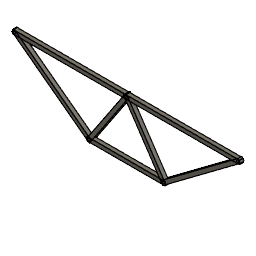
Truss_Assembly (Autodesk Fusion 360 design; units mm, degrees)
part number: 2026-09-01-19-27-21-433
Autodesk Fusion 360 part; units mm, degrees
sketch "Sketch1" plane through (0, 0, 0) normal (0, 0, 1) x (1, 0, 0)
  line L0 (-10.5, -10.5) -> (10.5, -10.5)
  line L1 (10.5, -10.5) -> (10.5, 10.5)
  line L2 (10.5, 10.5) -> (-10.5, 10.5)
  line L3 (-10.5, 10.5) -> (-10.5, -10.5)
sketch "Sketch2" plane through (0, 0, 0) normal (0, 0, 1) x (1, 0, 0)
  line L0 (-10.5, -10.5) -> (10.5, -10.5)
  line L1 (10.5, -10.5) -> (10.5, 10.5)
  line L2 (10.5, 10.5) -> (-10.5, 10.5)
  line L3 (-10.5, 10.5) -> (-10.5, -10.5)
sketch "Sketch3" plane through (0, 0, 0) normal (0, 0, 1) x (1, 0, 0)
  line L0 (-10.5, -10.5) -> (10.5, -10.5)
  line L1 (10.5, -10.5) -> (10.5, 10.5)
  line L2 (10.5, 10.5) -> (-10.5, 10.5)
  line L3 (-10.5, 10.5) -> (-10.5, -10.5)
sketch "Sketch4" plane through (0, 0, 0) normal (0, 0, 1) x (1, 0, 0)
  line L0 (-10.5, -10.5) -> (10.5, -10.5)
  line L1 (10.5, -10.5) -> (10.5, 10.5)
  line L2 (10.5, 10.5) -> (-10.5, 10.5)
  line L3 (-10.5, 10.5) -> (-10.5, -10.5)
sketch "Sketch5" plane through (0, 0, 0) normal (0, 0, 1) x (1, 0, 0)
  line L0 (-10.5, -10.5) -> (10.5, -10.5)
  line L1 (10.5, -10.5) -> (10.5, 10.5)
  line L2 (10.5, 10.5) -> (-10.5, 10.5)
  line L3 (-10.5, 10.5) -> (-10.5, -10.5)
sketch "Sketch6" plane through (0, 0, 0) normal (0, 0, 1) x (1, 0, 0)
  line L0 (-10.5, -10.5) -> (10.5, -10.5)
  line L1 (10.5, -10.5) -> (10.5, 10.5)
  line L2 (10.5, 10.5) -> (-10.5, 10.5)
  line L3 (-10.5, 10.5) -> (-10.5, -10.5)
sketch "Sketch7" plane through (0, 0, 0) normal (0, 0, 1) x (1, 0, 0)
  line L0 (-10.5, -10.5) -> (10.5, -10.5)
  line L1 (10.5, -10.5) -> (10.5, 10.5)
  line L2 (10.5, 10.5) -> (-10.5, 10.5)
  line L3 (-10.5, 10.5) -> (-10.5, -10.5)
sketch "Sketch8" plane through (0, 0, 0) normal (0, 0, 1) x (1, 0, 0)
  circle A0 centre (0, 0) radius 6.25
sketch "Sketch9" plane through (0, 0, 0) normal (0, 0, 1) x (1, 0, 0)
  circle A0 centre (600, 0) radius 6.25
sketch "Sketch10" plane through (0, 0, 0) normal (0, 0, 1) x (1, 0, 0)
  circle A0 centre (1200, 0) radius 6.25
sketch "Sketch11" plane through (0, 0, 0) normal (0, 0, 1) x (1, 0, 0)
  circle A0 centre (400, -299.3326) radius 6.25
sketch "Sketch12" plane through (0, 0, 0) normal (0, 0, 1) x (1, 0, 0)
  circle A0 centre (800, -299.3326) radius 6.25
sketch "Sketch13" plane through (0, 0, 0) normal (0, 0, 1) x (1, 0, 0)
  circle A0 centre (0, 0) radius 6.25
sketch "Sketch14" plane through (0, 0, 0) normal (0, 0, 1) x (1, 0, 0)
  circle A0 centre (0, 0) radius 6.25
sketch "Sketch15" plane through (0, 0, 0) normal (0, 0, 1) x (1, 0, 0)
  circle A0 centre (600, 0) radius 6.25
sketch "Sketch16" plane through (0, 0, 0) normal (0, 0, 1) x (1, 0, 0)
  circle A0 centre (600, 0) radius 6.25
sketch "Sketch17" plane through (0, 0, 0) normal (0, 0, 1) x (1, 0, 0)
  circle A0 centre (1200, 0) radius 6.25
sketch "Sketch18" plane through (0, 0, 0) normal (0, 0, 1) x (1, 0, 0)
  circle A0 centre (1200, 0) radius 6.25
sketch "Sketch19" plane through (0, 0, 0) normal (0, 0, 1) x (1, 0, 0)
  circle A0 centre (400, -299.3326) radius 6.25
sketch "Sketch20" plane through (0, 0, 0) normal (0, 0, 1) x (1, 0, 0)
  circle A0 centre (400, -299.3326) radius 6.25
sketch "Sketch21" plane through (0, 0, 0) normal (0, 0, 1) x (1, 0, 0)
  circle A0 centre (800, -299.3326) radius 6.25
sketch "Sketch22" plane through (0, 0, 0) normal (0, 0, 1) x (1, 0, 0)
  circle A0 centre (800, -299.3326) radius 6.25
sketch "Sketch23" plane through (0, 0, 0) normal (0, 0, 1) x (1, 0, 0)
  circle A0 centre (10.28, 0) radius 6.25
sketch "Sketch24" plane through (0, 0, 0) normal (0, 0, 1) x (1, 0, 0)
  circle A0 centre (10.28, 0) radius 6.25
sketch "Sketch25" plane through (0, 0, 0) normal (0, 0, 1) x (1, 0, 0)
  circle A0 centre (589.72, 0) radius 6.25
sketch "Sketch26" plane through (0, 0, 0) normal (0, 0, 1) x (1, 0, 0)
  circle A0 centre (589.72, 0) radius 6.25
sketch "Sketch27" plane through (0, 0, 0) normal (0, 0, 1) x (1, 0, 0)
  circle A0 centre (610.28, 0) radius 6.25
sketch "Sketch28" plane through (0, 0, 0) normal (0, 0, 1) x (1, 0, 0)
  circle A0 centre (610.28, 0) radius 6.25
sketch "Sketch29" plane through (0, 0, 0) normal (0, 0, 1) x (1, 0, 0)
  circle A0 centre (1189.72, 0) radius 6.25
sketch "Sketch30" plane through (0, 0, 0) normal (0, 0, 1) x (1, 0, 0)
  circle A0 centre (1189.72, 0) radius 6.25
sketch "Sketch31" plane through (0, 0, 0) normal (0, 0, 1) x (1, 0, 0)
  circle A0 centre (8.2306, -6.1592) radius 6.25
sketch "Sketch32" plane through (0, 0, 0) normal (0, 0, 1) x (1, 0, 0)
  circle A0 centre (8.2306, -6.1592) radius 6.25
sketch "Sketch33" plane through (0, 0, 0) normal (0, 0, 1) x (1, 0, 0)
  circle A0 centre (391.7694, -293.1734) radius 6.25
sketch "Sketch34" plane through (0, 0, 0) normal (0, 0, 1) x (1, 0, 0)
  circle A0 centre (391.7694, -293.1734) radius 6.25
sketch "Sketch35" plane through (0, 0, 0) normal (0, 0, 1) x (1, 0, 0)
  circle A0 centre (405.7111, -290.785) radius 6.25
sketch "Sketch36" plane through (0, 0, 0) normal (0, 0, 1) x (1, 0, 0)
  circle A0 centre (405.7111, -290.785) radius 6.25
sketch "Sketch37" plane through (0, 0, 0) normal (0, 0, 1) x (1, 0, 0)
  circle A0 centre (594.2889, -8.5476) radius 6.25
sketch "Sketch38" plane through (0, 0, 0) normal (0, 0, 1) x (1, 0, 0)
  circle A0 centre (594.2889, -8.5476) radius 6.25
sketch "Sketch39" plane through (0, 0, 0) normal (0, 0, 1) x (1, 0, 0)
  circle A0 centre (605.7111, -8.5476) radius 6.25
sketch "Sketch40" plane through (0, 0, 0) normal (0, 0, 1) x (1, 0, 0)
  circle A0 centre (605.7111, -8.5476) radius 6.25
sketch "Sketch41" plane through (0, 0, 0) normal (0, 0, 1) x (1, 0, 0)
  circle A0 centre (794.2889, -290.785) radius 6.25
sketch "Sketch42" plane through (0, 0, 0) normal (0, 0, 1) x (1, 0, 0)
  circle A0 centre (794.2889, -290.785) radius 6.25
sketch "Sketch43" plane through (0, 0, 0) normal (0, 0, 1) x (1, 0, 0)
  circle A0 centre (808.2306, -293.1734) radius 6.25
sketch "Sketch44" plane through (0, 0, 0) normal (0, 0, 1) x (1, 0, 0)
  circle A0 centre (808.2306, -293.1734) radius 6.25
sketch "Sketch45" plane through (0, 0, 0) normal (0, 0, 1) x (1, 0, 0)
  circle A0 centre (1191.7694, -6.1592) radius 6.25
sketch "Sketch46" plane through (0, 0, 0) normal (0, 0, 1) x (1, 0, 0)
  circle A0 centre (1191.7694, -6.1592) radius 6.25
sketch "Sketch47" plane through (0, 0, 0) normal (0, 0, 1) x (1, 0, 0)
  circle A0 centre (410.28, -299.3326) radius 6.25
sketch "Sketch48" plane through (0, 0, 0) normal (0, 0, 1) x (1, 0, 0)
  circle A0 centre (410.28, -299.3326) radius 6.25
sketch "Sketch49" plane through (0, 0, 0) normal (0, 0, 1) x (1, 0, 0)
  circle A0 centre (789.72, -299.3326) radius 6.25
sketch "Sketch50" plane through (0, 0, 0) normal (0, 0, 1) x (1, 0, 0)
  circle A0 centre (789.72, -299.3326) radius 6.25
sketch "Sketch51" plane through (0, 0, 0) normal (0, 0, 1) x (1, 0, 0)
  circle A0 centre (0, 0) radius 6.25
sketch "Sketch52" plane through (0, 0, 0) normal (0, 0, 1) x (1, 0, 0)
  circle A0 centre (0, 0) radius 6.25
sketch "Sketch53" plane through (0, 0, 0) normal (0, 0, 1) x (1, 0, 0)
  circle A0 centre (600, 0) radius 6.25
sketch "Sketch54" plane through (0, 0, 0) normal (0, 0, 1) x (1, 0, 0)
  circle A0 centre (600, 0) radius 6.25
sketch "Sketch55" plane through (0, 0, 0) normal (0, 0, 1) x (1, 0, 0)
  circle A0 centre (1200, 0) radius 6.25
sketch "Sketch56" plane through (0, 0, 0) normal (0, 0, 1) x (1, 0, 0)
  circle A0 centre (1200, 0) radius 6.25
sketch "Sketch57" plane through (0, 0, 0) normal (0, 0, 1) x (1, 0, 0)
  circle A0 centre (400, -299.3326) radius 6.25
sketch "Sketch58" plane through (0, 0, 0) normal (0, 0, 1) x (1, 0, 0)
  circle A0 centre (400, -299.3326) radius 6.25
sketch "Sketch59" plane through (0, 0, 0) normal (0, 0, 1) x (1, 0, 0)
  circle A0 centre (800, -299.3326) radius 6.25
sketch "Sketch60" plane through (0, 0, 0) normal (0, 0, 1) x (1, 0, 0)
  circle A0 centre (800, -299.3326) radius 6.25
sketch "Sketch61" plane through (0, 0, 0) normal (0, 0, 1) x (1, 0, 0)
  circle A0 centre (0, 0) radius 6.25
sketch "Sketch62" plane through (0, 0, 0) normal (0, 0, 1) x (1, 0, 0)
  circle A0 centre (600, 0) radius 6.25
sketch "Sketch63" plane through (0, 0, 0) normal (0, 0, 1) x (1, 0, 0)
  circle A0 centre (1200, 0) radius 6.25
sketch "Sketch64" plane through (0, 0, 0) normal (0, 0, 1) x (1, 0, 0)
  circle A0 centre (400, -299.3326) radius 6.25
sketch "Sketch65" plane through (0, 0, 0) normal (0, 0, 1) x (1, 0, 0)
  circle A0 centre (800, -299.3326) radius 6.25
sketch "Sketch66" plane through (0, 0, 0) normal (0, 0, 1) x (1, 0, 0)
  circle A0 centre (0, 0) radius 6.25
sketch "Sketch67" plane through (0, 0, 0) normal (0, 0, 1) x (1, 0, 0)
  circle A0 centre (600, 0) radius 6.25
sketch "Sketch68" plane through (0, 0, 0) normal (0, 0, 1) x (1, 0, 0)
  circle A0 centre (1200, 0) radius 6.25
sketch "Sketch69" plane through (0, 0, 0) normal (0, 0, 1) x (1, 0, 0)
  circle A0 centre (400, -299.3326) radius 6.25
sketch "Sketch70" plane through (0, 0, 0) normal (0, 0, 1) x (1, 0, 0)
  circle A0 centre (800, -299.3326) radius 6.25
ref_plane "WorkPlane1" through (0, 0, -20) normal (0, 0, 1) x (1, 0, 0)
sketch "Sketch71" plane through (0, 0, -20) normal (0, 0, 1) x (1, 0, 0)
  circle A0 centre (0, 0) radius 6.25
ref_plane "WorkPlane2" through (0, 0, -20) normal (0, 0, 1) x (1, 0, 0)
sketch "Sketch72" plane through (0, 0, -20) normal (0, 0, 1) x (1, 0, 0)
  circle A0 centre (600, 0) radius 6.25
ref_plane "WorkPlane3" through (0, 0, -20) normal (0, 0, 1) x (1, 0, 0)
sketch "Sketch73" plane through (0, 0, -20) normal (0, 0, 1) x (1, 0, 0)
  circle A0 centre (1200, 0) radius 6.25
ref_plane "WorkPlane4" through (0, 0, -20) normal (0, 0, 1) x (1, 0, 0)
sketch "Sketch74" plane through (0, 0, -20) normal (0, 0, 1) x (1, 0, 0)
  circle A0 centre (400, -299.3326) radius 6.25
ref_plane "WorkPlane5" through (0, 0, -20) normal (0, 0, 1) x (1, 0, 0)
sketch "Sketch75" plane through (0, 0, -20) normal (0, 0, 1) x (1, 0, 0)
  circle A0 centre (800, -299.3326) radius 6.25
ref_plane "WorkPlane6" through (0, 0, -50) normal (0, 0, 1) x (1, 0, 0)
sketch "Sketch76" plane through (0, 0, -50) normal (0, 0, 1) x (1, 0, 0)
  circle A0 centre (0, 0) radius 6.25
ref_plane "WorkPlane7" through (0, 0, -50) normal (0, 0, 1) x (1, 0, 0)
sketch "Sketch77" plane through (0, 0, -50) normal (0, 0, 1) x (1, 0, 0)
  circle A0 centre (600, 0) radius 6.25
ref_plane "WorkPlane8" through (0, 0, -50) normal (0, 0, 1) x (1, 0, 0)
sketch "Sketch78" plane through (0, 0, -50) normal (0, 0, 1) x (1, 0, 0)
  circle A0 centre (1200, 0) radius 6.25
ref_plane "WorkPlane9" through (0, 0, -50) normal (0, 0, 1) x (1, 0, 0)
sketch "Sketch79" plane through (0, 0, -50) normal (0, 0, 1) x (1, 0, 0)
  circle A0 centre (400, -299.3326) radius 6.25
ref_plane "WorkPlane10" through (0, 0, -50) normal (0, 0, 1) x (1, 0, 0)
sketch "Sketch80" plane through (0, 0, -50) normal (0, 0, 1) x (1, 0, 0)
  circle A0 centre (800, -299.3326) radius 6.25
sketch "Sketch81" plane through (0, 0, 0) normal (0, 0, 1) x (1, 0, 0)
  circle A0 centre (0, 0) radius 6.25
sketch "Sketch82" plane through (0, 0, 0) normal (0, 0, 1) x (1, 0, 0)
  circle A0 centre (600, 0) radius 6.25
sketch "Sketch83" plane through (0, 0, 0) normal (0, 0, 1) x (1, 0, 0)
  circle A0 centre (1200, 0) radius 6.25
sketch "Sketch84" plane through (0, 0, 0) normal (0, 0, 1) x (1, 0, 0)
  circle A0 centre (400, -299.3326) radius 6.25
sketch "Sketch85" plane through (0, 0, 0) normal (0, 0, 1) x (1, 0, 0)
  circle A0 centre (800, -299.3326) radius 6.25
sketch "Sketch86" plane through (0, 0, 0) normal (0, 0, 1) x (1, 0, 0)
  circle A0 centre (0, 0) radius 6.7276
sketch "Sketch87" plane through (0, 0, 0) normal (0, 0, 1) x (1, 0, 0)
  circle A0 centre (600, 0) radius 6.7276
sketch "Sketch88" plane through (0, 0, 0) normal (0, 0, 1) x (1, 0, 0)
  circle A0 centre (1200, 0) radius 6.7276
sketch "Sketch89" plane through (0, 0, 0) normal (0, 0, 1) x (1, 0, 0)
  circle A0 centre (400, -299.3326) radius 6.7276
sketch "Sketch90" plane through (0, 0, 0) normal (0, 0, 1) x (1, 0, 0)
  circle A0 centre (800, -299.3326) radius 6.7276
sketch "Sketch91" plane through (0, 0, 0) normal (0, 0, 1) x (1, 0, 0)
  line L0 (-10.5, -10.5) -> (10.5, -10.5)
  line L1 (10.5, -10.5) -> (10.5, 10.5)
  line L2 (10.5, 10.5) -> (-10.5, 10.5)
  line L3 (-10.5, 10.5) -> (-10.5, -10.5)
sketch "Sketch92" plane through (0, 0, 0) normal (0, 0, 1) x (1, 0, 0)
  line L0 (-10.5, -10.5) -> (10.5, -10.5)
  line L1 (10.5, -10.5) -> (10.5, 10.5)
  line L2 (10.5, 10.5) -> (-10.5, 10.5)
  line L3 (-10.5, 10.5) -> (-10.5, -10.5)
sketch "Sketch93" plane through (0, 0, 0) normal (0, 0, 1) x (1, 0, 0)
  line L0 (-10.5, -10.5) -> (10.5, -10.5)
  line L1 (10.5, -10.5) -> (10.5, 10.5)
  line L2 (10.5, 10.5) -> (-10.5, 10.5)
  line L3 (-10.5, 10.5) -> (-10.5, -10.5)
sketch "Sketch94" plane through (0, 0, 0) normal (0, 0, 1) x (1, 0, 0)
  line L0 (-10.5, -10.5) -> (10.5, -10.5)
  line L1 (10.5, -10.5) -> (10.5, 10.5)
  line L2 (10.5, 10.5) -> (-10.5, 10.5)
  line L3 (-10.5, 10.5) -> (-10.5, -10.5)
sketch "Sketch95" plane through (0, 0, 0) normal (0, 0, 1) x (1, 0, 0)
  line L0 (-10.5, -10.5) -> (10.5, -10.5)
  line L1 (10.5, -10.5) -> (10.5, 10.5)
  line L2 (10.5, 10.5) -> (-10.5, 10.5)
  line L3 (-10.5, 10.5) -> (-10.5, -10.5)
sketch "Sketch96" plane through (0, 0, 0) normal (0, 0, 1) x (1, 0, 0)
  line L0 (-10.5, -10.5) -> (10.5, -10.5)
  line L1 (10.5, -10.5) -> (10.5, 10.5)
  line L2 (10.5, 10.5) -> (-10.5, 10.5)
  line L3 (-10.5, 10.5) -> (-10.5, -10.5)
sketch "Sketch97" plane through (0, 0, 0) normal (0, 0, 1) x (1, 0, 0)
  line L0 (-10.5, -10.5) -> (10.5, -10.5)
  line L1 (10.5, -10.5) -> (10.5, 10.5)
  line L2 (10.5, 10.5) -> (-10.5, 10.5)
  line L3 (-10.5, 10.5) -> (-10.5, -10.5)
sketch "Sketch98" plane through (0, 0, 0) normal (0, 0, 1) x (1, 0, 0)
  line L0 (-10.5, -10.5) -> (10.5, -10.5)
  line L1 (10.5, -10.5) -> (10.5, 10.5)
  line L2 (10.5, 10.5) -> (-10.5, 10.5)
  line L3 (-10.5, 10.5) -> (-10.5, -10.5)
sketch "Sketch99" plane through (0, 0, 0) normal (0, 0, 1) x (1, 0, 0)
  line L0 (-10.5, -10.5) -> (10.5, -10.5)
  line L1 (10.5, -10.5) -> (10.5, 10.5)
  line L2 (10.5, 10.5) -> (-10.5, 10.5)
  line L3 (-10.5, 10.5) -> (-10.5, -10.5)
sketch "Sketch100" plane through (0, 0, 0) normal (0, 0, 1) x (1, 0, 0)
  line L0 (-10.5, -10.5) -> (10.5, -10.5)
  line L1 (10.5, -10.5) -> (10.5, 10.5)
  line L2 (10.5, 10.5) -> (-10.5, 10.5)
  line L3 (-10.5, 10.5) -> (-10.5, -10.5)
sketch "Sketch101" plane through (0, 0, 0) normal (0, 0, 1) x (1, 0, 0)
  line L0 (-10.5, -10.5) -> (10.5, -10.5)
  line L1 (10.5, -10.5) -> (10.5, 10.5)
  line L2 (10.5, 10.5) -> (-10.5, 10.5)
  line L3 (-10.5, 10.5) -> (-10.5, -10.5)
sketch "Sketch102" plane through (0, 0, 0) normal (0, 0, 1) x (1, 0, 0)
  line L0 (-10.5, -10.5) -> (10.5, -10.5)
  line L1 (10.5, -10.5) -> (10.5, 10.5)
  line L2 (10.5, 10.5) -> (-10.5, 10.5)
  line L3 (-10.5, 10.5) -> (-10.5, -10.5)
sketch "Sketch103" plane through (0, 0, 0) normal (0, 0, 1) x (1, 0, 0)
  line L0 (-10.5, -10.5) -> (10.5, -10.5)
  line L1 (10.5, -10.5) -> (10.5, 10.5)
  line L2 (10.5, 10.5) -> (-10.5, 10.5)
  line L3 (-10.5, 10.5) -> (-10.5, -10.5)
sketch "Sketch104" plane through (0, 0, 0) normal (0, 0, 1) x (1, 0, 0)
  line L0 (-10.5, -10.5) -> (10.5, -10.5)
  line L1 (10.5, -10.5) -> (10.5, 10.5)
  line L2 (10.5, 10.5) -> (-10.5, 10.5)
  line L3 (-10.5, 10.5) -> (-10.5, -10.5)
sketch "Sketch105" plane through (0, 0, 0) normal (0, 0, 1) x (1, 0, 0)
  circle A0 centre (0, 0) radius 6.25
sketch "Sketch106" plane through (0, 0, 0) normal (0, 0, 1) x (1, 0, 0)
  circle A0 centre (600, 0) radius 6.25
sketch "Sketch107" plane through (0, 0, 0) normal (0, 0, 1) x (1, 0, 0)
  circle A0 centre (1200, 0) radius 6.25
sketch "Sketch108" plane through (0, 0, 0) normal (0, 0, 1) x (1, 0, 0)
  circle A0 centre (400, -299.3326) radius 6.25
sketch "Sketch115" plane through (0, 0, 0) normal (0, 0, 1) x (1, 0, 0)
  circle A0 centre (0, 0) radius 6.25
sketch "Sketch116" plane through (0, 0, 0) normal (0, 0, 1) x (1, 0, 0)
  circle A0 centre (600, 0) radius 6.25
sketch "Sketch117" plane through (0, 0, 0) normal (0, 0, 1) x (1, 0, 0)
  circle A0 centre (1200, 0) radius 6.25
sketch "Sketch118" plane through (0, 0, 0) normal (0, 0, 1) x (1, 0, 0)
  circle A0 centre (400, -299.3326) radius 6.25
sketch "Sketch119" plane through (0, 0, 0) normal (0, 0, 1) x (1, 0, 0)
  circle A0 centre (800, -299.3326) radius 6.25
sketch "Sketch120" plane through (0, 0, 0) normal (0, 0, 1) x (1, 0, 0)
  line L0 (-10.5, -10.5) -> (10.5, -10.5)
  line L1 (10.5, -10.5) -> (10.5, 10.5)
  line L2 (10.5, 10.5) -> (-10.5, 10.5)
  line L3 (-10.5, 10.5) -> (-10.5, -10.5)
sketch "Sketch121" plane through (0, 0, 0) normal (0, 0, 1) x (1, 0, 0)
  circle A0 centre (-590.0371, 146.3512) radius 6.25
sketch "Sketch122" plane through (0, 0, 0) normal (0, 0, 1) x (1, 0, 0)
  circle A0 centre (0, 139.1663) radius 6.25
sketch "Sketch126" plane through (0, 0, 0) normal (0, 0, 1) x (1, 0, 0)
  circle A0 centre (-600, 149.6663) radius 6.25
sketch "Sketch127" plane through (0, 0, 0) normal (0, 0, 1) x (1, 0, 0)
  circle A0 centre (0, 149.6663) radius 6.25
sketch "Sketch128" plane through (0, 0, 0) normal (0, 0, 1) x (1, 0, 0)
  circle A0 centre (600, 149.6663) radius 6.25
sketch "Sketch129" plane through (0, 0, 0) normal (0, 0, 1) x (1, 0, 0)
  circle A0 centre (-200, -149.6663) radius 6.25
sketch "Sketch130" plane through (0, 0, 0) normal (0, 0, 1) x (1, 0, 0)
  circle A0 centre (200, -149.6663) radius 6.25
sketch "Sketch131" plane through (0, 0, 0) normal (0, 0, 1) x (1, 0, 0)
  circle A0 centre (8.4067, -6.291) radius 6.25
sketch "Sketch132" plane through (0, 0, 0) normal (0, 0, 1) x (1, 0, 0)
  circle A0 centre (8.4067, -6.291) radius 6.25
sketch "Sketch133" plane through (0, 0, 0) normal (0, 0, 1) x (1, 0, 0)
  circle A0 centre (391.5933, -293.0416) radius 6.25
sketch "Sketch134" plane through (0, 0, 0) normal (0, 0, 1) x (1, 0, 0)
  circle A0 centre (391.5933, -293.0416) radius 6.25
sketch "Sketch135" plane through (0, 0, 0) normal (0, 0, 1) x (1, 0, 0)
  circle A0 centre (405.8333, -290.6021) radius 6.25
sketch "Sketch136" plane through (0, 0, 0) normal (0, 0, 1) x (1, 0, 0)
  circle A0 centre (405.8333, -290.6021) radius 6.25
sketch "Sketch137" plane through (0, 0, 0) normal (0, 0, 1) x (1, 0, 0)
  circle A0 centre (594.1667, -8.7305) radius 6.25
sketch "Sketch138" plane through (0, 0, 0) normal (0, 0, 1) x (1, 0, 0)
  circle A0 centre (594.1667, -8.7305) radius 6.25
sketch "Sketch139" plane through (0, 0, 0) normal (0, 0, 1) x (1, 0, 0)
  circle A0 centre (605.8333, -8.7305) radius 6.25
sketch "Sketch140" plane through (0, 0, 0) normal (0, 0, 1) x (1, 0, 0)
  circle A0 centre (605.8333, -8.7305) radius 6.25
sketch "Sketch141" plane through (0, 0, 0) normal (0, 0, 1) x (1, 0, 0)
  circle A0 centre (794.1667, -290.6021) radius 6.25
sketch "Sketch142" plane through (0, 0, 0) normal (0, 0, 1) x (1, 0, 0)
  circle A0 centre (794.1667, -290.6021) radius 6.25
sketch "Sketch143" plane through (0, 0, 0) normal (0, 0, 1) x (1, 0, 0)
  circle A0 centre (808.4067, -293.0416) radius 6.25
sketch "Sketch144" plane through (0, 0, 0) normal (0, 0, 1) x (1, 0, 0)
  circle A0 centre (808.4067, -293.0416) radius 6.25
sketch "Sketch145" plane through (0, 0, 0) normal (0, 0, 1) x (1, 0, 0)
  circle A0 centre (1191.5933, -6.291) radius 6.25
sketch "Sketch146" plane through (0, 0, 0) normal (0, 0, 1) x (1, 0, 0)
  circle A0 centre (1191.5933, -6.291) radius 6.25
sketch "Sketch147" plane through (0, 0, 0) normal (0, 0, 1) x (1, 0, 0)
  circle A0 centre (410.5, -299.3326) radius 6.25
sketch "Sketch148" plane through (0, 0, 0) normal (0, 0, 1) x (1, 0, 0)
  circle A0 centre (410.5, -299.3326) radius 6.25
sketch "Sketch149" plane through (0, 0, 0) normal (0, 0, 1) x (1, 0, 0)
  circle A0 centre (789.5, -299.3326) radius 6.25
sketch "Sketch150" plane through (0, 0, 0) normal (0, 0, 1) x (1, 0, 0)
  circle A0 centre (789.5, -299.3326) radius 6.25
sketch "Sketch151" plane through (0, 0, 0) normal (0, 0, 1) x (1, 0, 0)
  circle A0 centre (-600, 0) radius 6.25
sketch "Sketch152" plane through (0, 0, 0) normal (0, 0, 1) x (1, 0, 0)
  circle A0 centre (0, 0) radius 6.25
sketch "Sketch153" plane through (0, 0, 0) normal (0, 0, 1) x (1, 0, 0)
  circle A0 centre (600, 0) radius 6.25
sketch "Sketch166" plane through (0, 0, 0) normal (0, 0, 1) x (1, 0, 0)
  circle A0 centre (-600, 149.6663) radius 6.25
sketch "Sketch167" plane through (0, 0, 0) normal (0, 0, 1) x (1, 0, 0)
  circle A0 centre (0, 149.6663) radius 6.25
sketch "Sketch168" plane through (0, 0, 0) normal (0, 0, 1) x (1, 0, 0)
  circle A0 centre (600, 149.6663) radius 6.25
sketch "Sketch169" plane through (0, 0, 0) normal (0, 0, 1) x (1, 0, 0)
  circle A0 centre (-200, -149.6663) radius 6.25
sketch "Sketch170" plane through (0, 0, 0) normal (0, 0, 1) x (1, 0, 0)
  circle A0 centre (200, -149.6663) radius 6.25
sketch "Sketch171" plane through (0, 0, 0) normal (0, 0, 1) x (1, 0, 0)
  line L0 (-10.5, -10.5) -> (10.5, -10.5)
  line L1 (10.5, -10.5) -> (10.5, 10.5)
  line L2 (10.5, 10.5) -> (-10.5, 10.5)
  line L3 (-10.5, 10.5) -> (-10.5, -10.5)
sketch "Sketch172" plane through (0, 0, 0) normal (0, 0, 1) x (1, 0, 0)
  line L0 (-10.5, -10.5) -> (10.5, -10.5)
  line L1 (10.5, -10.5) -> (10.5, 10.5)
  line L2 (10.5, 10.5) -> (-10.5, 10.5)
  line L3 (-10.5, 10.5) -> (-10.5, -10.5)
sketch "Sketch173" plane through (0, 0, 0) normal (0, 0, 1) x (1, 0, 0)
  line L0 (-10.5, -10.5) -> (10.5, -10.5)
  line L1 (10.5, -10.5) -> (10.5, 10.5)
  line L2 (10.5, 10.5) -> (-10.5, 10.5)
  line L3 (-10.5, 10.5) -> (-10.5, -10.5)
sketch "Sketch174" plane through (0, 0, 0) normal (0, 0, 1) x (1, 0, 0)
  line L0 (-10.5, -10.5) -> (10.5, -10.5)
  line L1 (10.5, -10.5) -> (10.5, 10.5)
  line L2 (10.5, 10.5) -> (-10.5, 10.5)
  line L3 (-10.5, 10.5) -> (-10.5, -10.5)
sketch "Sketch175" plane through (0, 0, 0) normal (0, 0, 1) x (1, 0, 0)
  line L0 (-10.5, -10.5) -> (10.5, -10.5)
  line L1 (10.5, -10.5) -> (10.5, 10.5)
  line L2 (10.5, 10.5) -> (-10.5, 10.5)
  line L3 (-10.5, 10.5) -> (-10.5, -10.5)
sketch "Sketch176" plane through (0, 0, 0) normal (0, 0, 1) x (1, 0, 0)
  line L0 (-10.5, -10.5) -> (10.5, -10.5)
  line L1 (10.5, -10.5) -> (10.5, 10.5)
  line L2 (10.5, 10.5) -> (-10.5, 10.5)
  line L3 (-10.5, 10.5) -> (-10.5, -10.5)
sketch "Sketch177" plane through (0, 0, 0) normal (0, 0, 1) x (1, 0, 0)
  circle A0 centre (-610.5, 0) radius 6.25
sketch "Sketch178" plane through (0, 0, 0) normal (0, 0, 1) x (1, 0, 0)
  circle A0 centre (-610.5, 0) radius 6.25
sketch "Sketch179" plane through (0, 0, 0) normal (0, 0, 1) x (1, 0, 0)
  circle A0 centre (0, 0) radius 6.25
sketch "Sketch180" plane through (0, 0, 0) normal (0, 0, 1) x (1, 0, 0)
  circle A0 centre (0, 0) radius 6.25
sketch "Sketch181" plane through (0, 0, 0) normal (0, 0, 1) x (1, 0, 0)
  circle A0 centre (610.5, 0) radius 6.25
sketch "Sketch182" plane through (0, 0, 0) normal (0, 0, 1) x (1, 0, 0)
  circle A0 centre (610.5, 0) radius 6.25
sketch "Sketch183" plane through (0, 0, 0) normal (0, 0, 1) x (1, 0, 0)
  circle A0 centre (-210.5, -299.33) radius 6.25
sketch "Sketch184" plane through (0, 0, 0) normal (0, 0, 1) x (1, 0, 0)
  circle A0 centre (-210.5, -299.33) radius 6.25
sketch "Sketch185" plane through (0, 0, 0) normal (0, 0, 1) x (1, 0, 0)
  circle A0 centre (210.5, -299.33) radius 6.25
sketch "Sketch186" plane through (0, 0, 0) normal (0, 0, 1) x (1, 0, 0)
  circle A0 centre (210.5, -299.33) radius 6.25
sketch "Sketch187" plane through (0, 0, 0) normal (0, 0, 1) x (1, 0, 0)
  circle A0 centre (-610.5, 0) radius 6.25
sketch "Sketch188" plane through (0, 0, 0) normal (0, 0, 1) x (1, 0, 0)
  circle A0 centre (-610.5, 0) radius 6.25
sketch "Sketch189" plane through (0, 0, 0) normal (0, 0, 1) x (1, 0, 0)
  circle A0 centre (0, 0) radius 6.25
sketch "Sketch190" plane through (0, 0, 0) normal (0, 0, 1) x (1, 0, 0)
  circle A0 centre (0, 0) radius 6.25
sketch "Sketch191" plane through (0, 0, 0) normal (0, 0, 1) x (1, 0, 0)
  circle A0 centre (610.5, 0) radius 6.25
sketch "Sketch192" plane through (0, 0, 0) normal (0, 0, 1) x (1, 0, 0)
  circle A0 centre (610.5, 0) radius 6.25
sketch "Sketch193" plane through (0, 0, 0) normal (0, 0, 1) x (1, 0, 0)
  circle A0 centre (-210.5, -299.33) radius 6.25
sketch "Sketch194" plane through (0, 0, 0) normal (0, 0, 1) x (1, 0, 0)
  circle A0 centre (-210.5, -299.33) radius 6.25
sketch "Sketch195" plane through (0, 0, 0) normal (0, 0, 1) x (1, 0, 0)
  circle A0 centre (210.5, -299.33) radius 6.25
sketch "Sketch196" plane through (0, 0, 0) normal (0, 0, 1) x (1, 0, 0)
  circle A0 centre (210.5, -299.33) radius 6.25
sketch "Sketch197" plane through (0, 0, 0) normal (0, 0, 1) x (1, 0, 0)
  line L0 (-10.5, -10.5) -> (10.5, -10.5)
  line L1 (10.5, -10.5) -> (10.5, 10.5)
  line L2 (10.5, 10.5) -> (-10.5, 10.5)
  line L3 (-10.5, 10.5) -> (-10.5, -10.5)
sketch "Sketch198" plane through (0, 0, 0) normal (0, 0, 1) x (1, 0, 0)
  line L0 (-10.5, -10.5) -> (10.5, -10.5)
  line L1 (10.5, -10.5) -> (10.5, 10.5)
  line L2 (10.5, 10.5) -> (-10.5, 10.5)
  line L3 (-10.5, 10.5) -> (-10.5, -10.5)
sketch "Sketch199" plane through (0, 0, 0) normal (0, 0, 1) x (1, 0, 0)
  line L0 (-10.5, -10.5) -> (10.5, -10.5)
  line L1 (10.5, -10.5) -> (10.5, 10.5)
  line L2 (10.5, 10.5) -> (-10.5, 10.5)
  line L3 (-10.5, 10.5) -> (-10.5, -10.5)
sketch "Sketch200" plane through (0, 0, 0) normal (0, 0, 1) x (1, 0, 0)
  line L0 (-10.5, -10.5) -> (10.5, -10.5)
  line L1 (10.5, -10.5) -> (10.5, 10.5)
  line L2 (10.5, 10.5) -> (-10.5, 10.5)
  line L3 (-10.5, 10.5) -> (-10.5, -10.5)
sketch "Sketch201" plane through (0, 0, 0) normal (0, 0, 1) x (1, 0, 0)
  line L0 (-10.5, -10.5) -> (10.5, -10.5)
  line L1 (10.5, -10.5) -> (10.5, 10.5)
  line L2 (10.5, 10.5) -> (-10.5, 10.5)
  line L3 (-10.5, 10.5) -> (-10.5, -10.5)
sketch "Sketch202" plane through (0, 0, 0) normal (0, 0, 1) x (1, 0, 0)
  line L0 (-10.5, -10.5) -> (10.5, -10.5)
  line L1 (10.5, -10.5) -> (10.5, 10.5)
  line L2 (10.5, 10.5) -> (-10.5, 10.5)
  line L3 (-10.5, 10.5) -> (-10.5, -10.5)
sketch "Sketch203" plane through (0, 0, 0) normal (0, 0, 1) x (1, 0, 0)
  circle A0 centre (-600, 0) radius 6.25
sketch "Sketch204" plane through (0, 0, 0) normal (0, 0, 1) x (1, 0, 0)
  circle A0 centre (-600, 0) radius 6.25
sketch "Sketch205" plane through (0, 0, 0) normal (0, 0, 1) x (1, 0, 0)
  circle A0 centre (0, 0) radius 6.25
sketch "Sketch206" plane through (0, 0, 0) normal (0, 0, 1) x (1, 0, 0)
  circle A0 centre (0, 0) radius 6.25
sketch "Sketch207" plane through (0, 0, 0) normal (0, 0, 1) x (1, 0, 0)
  circle A0 centre (600, 0) radius 6.25
sketch "Sketch208" plane through (0, 0, 0) normal (0, 0, 1) x (1, 0, 0)
  circle A0 centre (600, 0) radius 6.25
sketch "Sketch209" plane through (0, 0, 0) normal (0, 0, 1) x (1, 0, 0)
  circle A0 centre (-200, -299.3326) radius 6.25
sketch "Sketch210" plane through (0, 0, 0) normal (0, 0, 1) x (1, 0, 0)
  circle A0 centre (-200, -299.3326) radius 6.25
sketch "Sketch211" plane through (0, 0, 0) normal (0, 0, 1) x (1, 0, 0)
  circle A0 centre (200, -299.3326) radius 6.25
sketch "Sketch212" plane through (0, 0, 0) normal (0, 0, 1) x (1, 0, 0)
  circle A0 centre (200, -299.3326) radius 6.25
sketch "Sketch213" plane through (0, 0, 0) normal (0, 0, 1) x (1, 0, 0)
  circle A0 centre (-610.5, 0) radius 6.25
sketch "Sketch214" plane through (0, 0, 0) normal (0, 0, 1) x (1, 0, 0)
  circle A0 centre (-610.5, 0) radius 6.25
sketch "Sketch215" plane through (0, 0, 0) normal (0, 0, 1) x (1, 0, 0)
  circle A0 centre (0, 0) radius 6.25
sketch "Sketch216" plane through (0, 0, 0) normal (0, 0, 1) x (1, 0, 0)
  circle A0 centre (0, 0) radius 6.25
sketch "Sketch217" plane through (0, 0, 0) normal (0, 0, 1) x (1, 0, 0)
  circle A0 centre (610.5, 0) radius 6.25
sketch "Sketch218" plane through (0, 0, 0) normal (0, 0, 1) x (1, 0, 0)
  circle A0 centre (610.5, 0) radius 6.25
sketch "Sketch219" plane through (0, 0, 0) normal (0, 0, 1) x (1, 0, 0)
  circle A0 centre (-210.5, -299.33) radius 6.25
sketch "Sketch220" plane through (0, 0, 0) normal (0, 0, 1) x (1, 0, 0)
  circle A0 centre (-210.5, -299.33) radius 6.25
sketch "Sketch221" plane through (0, 0, 0) normal (0, 0, 1) x (1, 0, 0)
  circle A0 centre (210.5, -299.33) radius 6.25
sketch "Sketch222" plane through (0, 0, 0) normal (0, 0, 1) x (1, 0, 0)
  circle A0 centre (210.5, -299.33) radius 6.25
sketch "Sketch223" plane through (0, 0, 0) normal (0, 0, 1) x (1, 0, 0)
  line L0 (-10.5, -10.5) -> (10.5, -10.5)
  line L1 (10.5, -10.5) -> (10.5, 10.5)
  line L2 (10.5, 10.5) -> (-10.5, 10.5)
  line L3 (-10.5, 10.5) -> (-10.5, -10.5)
extrude "Extrude222" add sketch "Sketch223" along normal blind 1220.56 makes body 1
move_body "Move48" bodies 1 to x (0, -1, 0) y (0, 0, -1) z (1, 0, 0) at (-610.28, 0, 0)
sketch "Sketch224" plane through (0, 0, 0) normal (0, 0, 1) x (1, 0, 0)
  line L0 (-10.5, -10.5) -> (10.5, -10.5)
  line L1 (10.5, -10.5) -> (10.5, 10.5)
  line L2 (10.5, 10.5) -> (-10.5, 10.5)
  line L3 (-10.5, 10.5) -> (-10.5, -10.5)
extrude "Extrude223" add sketch "Sketch224" along normal blind 520.1598 separate body makes body 2
move_body "Move49" bodies 2 to x (-0.599145, -0.800641, 0) y (0, 0, -1) z (0.800641, -0.599145, 0) at (-608.2306, 6.1592, 0)
sketch "Sketch225" plane through (0, 0, 0) normal (0, 0, 1) x (1, 0, 0)
  line L0 (-10.5, -10.5) -> (10.5, -10.5)
  line L1 (10.5, -10.5) -> (10.5, 10.5)
  line L2 (10.5, 10.5) -> (-10.5, 10.5)
  line L3 (-10.5, 10.5) -> (-10.5, -10.5)
extrude "Extrude224" add sketch "Sketch225" along normal blind 380.56 separate body makes body 3
move_body "Move50" bodies 3 to x (0.831479, -0.555556, 0) y (0, 0, -1) z (0.555556, 0.831479, 0) at (-205.7111, -307.8802, 0)
sketch "Sketch226" plane through (0, 0, 0) normal (0, 0, 1) x (1, 0, 0)
  line L0 (-10.5, -10.5) -> (10.5, -10.5)
  line L1 (10.5, -10.5) -> (10.5, 10.5)
  line L2 (10.5, 10.5) -> (-10.5, 10.5)
  line L3 (-10.5, 10.5) -> (-10.5, -10.5)
extrude "Extrude225" add sketch "Sketch226" along normal blind 380.56 separate body makes body 4
move_body "Move51" bodies 4 to x (-0.831479, -0.555556, 0) y (0, 0, -1) z (0.555556, -0.831479, 0) at (-5.7111, 8.5476, 0)
sketch "Sketch227" plane through (0, 0, 0) normal (0, 0, 1) x (1, 0, 0)
  line L0 (-10.5, -10.5) -> (10.5, -10.5)
  line L1 (10.5, -10.5) -> (10.5, 10.5)
  line L2 (10.5, 10.5) -> (-10.5, 10.5)
  line L3 (-10.5, 10.5) -> (-10.5, -10.5)
extrude "Extrude226" add sketch "Sketch227" along normal blind 520.1598 separate body makes body 5
move_body "Move52" bodies 5 to x (0.599145, -0.800641, 0) y (0, 0, -1) z (0.800641, 0.599145, 0) at (191.7694, -305.4918, 0)
sketch "Sketch228" plane through (0, 0, 0) normal (0, 0, 1) x (1, 0, 0)
  line L0 (-10.5, -10.5) -> (10.5, -10.5)
  line L1 (10.5, -10.5) -> (10.5, 10.5)
  line L2 (10.5, 10.5) -> (-10.5, 10.5)
  line L3 (-10.5, 10.5) -> (-10.5, -10.5)
extrude "Extrude227" add sketch "Sketch228" along normal blind 420.56 separate body makes body 6
move_body "Move53" bodies 6 to x (0, -1, 0) y (0, 0, -1) z (1, 0, 0) at (-210.28, -299.3326, 0)
sketch "Sketch229" plane through (0, 0, 0) normal (0, 0, 1) x (1, 0, 0)
  circle A0 centre (-600, 0) radius 6.25
extrude "Extrude228" add sketch "Sketch229" along normal mid plane 21 separate body makes body 7
sketch "Sketch230" plane through (0, 0, 0) normal (0, 0, 1) x (1, 0, 0)
  circle A0 centre (-600, 0) radius 6.25
extrude "Extrude229" cut sketch "Sketch230" along normal mid plane 21 bodies 1 2 3 4 5 6
sketch "Sketch231" plane through (0, 0, 0) normal (0, 0, 1) x (1, 0, 0)
  circle A0 centre (0, 0) radius 6.25
extrude "Extrude230" add sketch "Sketch231" along normal mid plane 21 separate body makes body 8
sketch "Sketch232" plane through (0, 0, 0) normal (0, 0, 1) x (1, 0, 0)
  circle A0 centre (0, 0) radius 6.25
extrude "Extrude231" cut sketch "Sketch232" along normal mid plane 21 bodies 1 2 3 4 5 6
sketch "Sketch233" plane through (0, 0, 0) normal (0, 0, 1) x (1, 0, 0)
  circle A0 centre (600, 0) radius 6.25
extrude "Extrude232" add sketch "Sketch233" along normal mid plane 21 separate body makes body 9
sketch "Sketch234" plane through (0, 0, 0) normal (0, 0, 1) x (1, 0, 0)
  circle A0 centre (600, 0) radius 6.25
extrude "Extrude233" cut sketch "Sketch234" along normal mid plane 21 bodies 1 2 3 4 5 6
sketch "Sketch235" plane through (0, 0, 0) normal (0, 0, 1) x (1, 0, 0)
  circle A0 centre (-200, -299.3326) radius 6.25
extrude "Extrude234" add sketch "Sketch235" along normal mid plane 21 separate body makes body 10
sketch "Sketch236" plane through (0, 0, 0) normal (0, 0, 1) x (1, 0, 0)
  circle A0 centre (-200, -299.3326) radius 6.25
extrude "Extrude235" cut sketch "Sketch236" along normal mid plane 21 bodies 1 2 3 4 5 6
sketch "Sketch237" plane through (0, 0, 0) normal (0, 0, 1) x (1, 0, 0)
  circle A0 centre (200, -299.3326) radius 6.25
extrude "Extrude236" add sketch "Sketch237" along normal mid plane 21 separate body makes body 11
sketch "Sketch238" plane through (0, 0, 0) normal (0, 0, 1) x (1, 0, 0)
  circle A0 centre (200, -299.3326) radius 6.25
extrude "Extrude237" cut sketch "Sketch238" along normal mid plane 21 bodies 1 2 3 4 5 6
sketch "Sketch154" plane through (0, 0, 0) normal (0, 0, 1) x (1, 0, 0)
  circle A0 centre (-200, -299.3326) radius 6.25
sketch "Sketch155" plane through (0, 0, 0) normal (0, 0, 1) x (1, 0, 0)
  circle A0 centre (200, -299.3326) radius 6.25
sketch "Sketch156" plane through (0, 0, 0) normal (0, 0, 1) x (1, 0, 0)
  circle A0 centre (9.9629, -3.3151) radius 6.25
sketch "Sketch157" plane through (0, 0, 0) normal (0, 0, 1) x (1, 0, 0)
  circle A0 centre (600, -10.5) radius 6.25
sketch "Sketch158" plane through (0, 0, 0) normal (0, 0, 1) x (1, 0, 0)
  circle A0 centre (1190.0371, -3.3151) radius 6.25
sketch "Sketch159" plane through (0, 0, 0) normal (0, 0, 1) x (1, 0, 0)
  circle A0 centre (404.9003, -290.0462) radius 6.25
sketch "Sketch160" plane through (0, 0, 0) normal (0, 0, 1) x (1, 0, 0)
  circle A0 centre (795.0997, -290.0462) radius 6.25
sketch "Sketch161" plane through (0, 0, 0) normal (0, 0, 1) x (1, 0, 0)
  circle A0 centre (-6.291, 10.5) radius 6.25
sketch "Sketch162" plane through (0, 0, 0) normal (0, 0, 1) x (1, 0, 0)
  circle A0 centre (1206.291, 10.5) radius 6.25
sketch "Sketch163" plane through (0, 0, 0) normal (0, 0, 1) x (1, 0, 0)
  circle A0 centre (600, 10.5) radius 6.25
sketch "Sketch164" plane through (0, 0, 0) normal (0, 0, 1) x (1, 0, 0)
  circle A0 centre (397.903, -309.8326) radius 6.25
sketch "Sketch165" plane through (0, 0, 0) normal (0, 0, 1) x (1, 0, 0)
  circle A0 centre (802.097, -309.8326) radius 6.25
extrude "Extrude122" [suppressed]
sketch "Sketch123" plane through (0, 0, 0) normal (0, 0, 1) x (1, 0, 0)
  circle A0 centre (590.0371, 146.3512) radius 6.25
extrude "Extrude123" [suppressed]
sketch "Sketch124" plane through (0, 0, 0) normal (0, 0, 1) x (1, 0, 0)
  circle A0 centre (-195.0997, -140.3799) radius 6.25
extrude "Extrude124" [suppressed]
sketch "Sketch125" plane through (0, 0, 0) normal (0, 0, 1) x (1, 0, 0)
  circle A0 centre (195.0997, -140.3799) radius 6.25
extrude "Extrude125" [suppressed]
sketch "Sketch109" plane through (0, 0, 0) normal (0, 0, 1) x (1, 0, 0)
  circle A0 centre (800, -299.3326) radius 6.25
sketch "Sketch110" plane through (0, 0, 0) normal (0, 0, 1) x (1, 0, 0)
  circle A0 centre (-600, 149.6663) radius 6.25
extrude "Extrude110" [suppressed]
sketch "Sketch111" plane through (0, 0, 0) normal (0, 0, 1) x (1, 0, 0)
  circle A0 centre (0, 149.6663) radius 6.25
extrude "Extrude111" [suppressed]
sketch "Sketch112" plane through (0, 0, 0) normal (0, 0, 1) x (1, 0, 0)
  circle A0 centre (600, 149.6663) radius 6.25
extrude "Extrude112" [suppressed]
sketch "Sketch113" plane through (0, 0, 0) normal (0, 0, 1) x (1, 0, 0)
  circle A0 centre (-200, -149.6663) radius 6.25
extrude "Extrude113" [suppressed]
sketch "Sketch114" plane through (0, 0, 0) normal (0, 0, 1) x (1, 0, 0)
  circle A0 centre (200, -149.6663) radius 6.25
extrude "Extrude114" [suppressed]
named bodies: "Pin_B", "Pin_E", "Pin_A", "Pin_D", "Pin_C", "Member_AB", "Member_BD", "Member_DE", "Member_EC", "Member_CA", "Member_DC"
